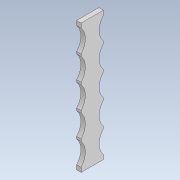
# Autodesk Inventor part: aileron_traverse
Saved by Autodesk Inventor 2020 (Build 240168000, 168)
## iProperties
Created: 2020-09-10
Part Number: aileron_traverse
Material: Generic
Document SubType Name: Modeling
Designer: Admin
Density: 1 g/cm^3
Appearance: Default
Author: Admin
Autodesk Inventor part; units mm, degrees
ref_plane "YZ Plane" through (0, 0, 0) normal (1, 0, 0) x (0, 1, 0)
ref_plane "XZ Plane" through (0, 0, 0) normal (0, 1, 0) x (-1, 0, 0)
ref_plane "XY Plane" through (0, 0, 0) normal (0, 0, 1) x (1, 0, 0)
sketch "Sketch1" plane through (0, 0, 0) normal (0, 1, 0) x (-1, 0, 0)
  line L0 (0, 0) -> (2, 0)
  line L1 (2, 0) -> (2, -10)
  line L2 (2, -10) -> (0, -10)
  line L3 (0, -10) -> (0, 0)
  dimension "d0" = 10
  dimension "d1" = 2
  constraints: 8 end point, 2 parallel, 1 horizontal, 1 perpendicular
  measures "d0" distance of L0.end L1.end
  measures "d1" distance of L1.end L2.end
extrude "Extrusion1" add sketch "Sketch1" along normal blind 58
sketch "Sketch3" plane through (0, 0, 0) normal (1, 0, 0) x (0, 0, -1)
  line L0 (0, 58) -> (10, 58) projected
  line L1 (10, 56) -> (10, 46)
  arc A0 (10, 56) -> (10, 46) centre (15.5902, 51) ccw
  line L2 (10, 0) -> (10, 58) projected
  line L3 (0, 56) -> (0, 46)
  arc A1 (0, 46) -> (0, 56) centre (-5.5902, 51) ccw
  line L4 (0, 0) -> (0, 58) projected
  dimension "d12" = 10
  dimension "d13" = 2
  dimension "d14" = 7.5
  dimension "d15" = 10
  dimension "d16" = 7.5
  dimension "d17" = 2
  constraints: 4 end point, 4 point on circle, 2 centre point, 2 point on line, 2 vertical
  measures "d12" distance of L1.start L1.end
  measures "d13" distance from line of L1.start L0
  measures "d14" radius of A0
  measures "d15" distance of L3.start L3.end
  measures "d16" radius of A1
  measures "d17" distance from line of L0 L3.start
extrude "Extrusion3" cut sketch "Sketch3" against normal blind 58
pattern_linear "Rectangular Pattern1" count 5 spacing 11 along (0, -1, 0) of "Extrusion3"
body "Solid1"
